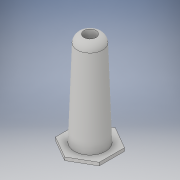
# Autodesk Inventor part: insert
Saved by Autodesk Inventor 2017 (Build 210142000, 142)
## iProperties
Created: 2017-08-01
Part Number: insert
Material: Generic
Document SubType Name: Modeling
Designer: Mitch
Density: 1 g/cm^3
Appearance: Default
Author: Mitch
Autodesk Inventor part; units mm, degrees
ref_plane "YZ Plane" through (0, 0, 0) normal (1, 0, 0) x (0, 1, 0)
ref_plane "XZ Plane" through (0, 0, 0) normal (0, 1, 0) x (-1, 0, 0)
sketch "Sketch1" plane through (0, 0, 0) normal (0, 1, 0) x (-1, 0, 0)
  line L0 (0, -10.2653) -> (-8.89, -5.1326)
  line L1 (-8.89, -5.1326) -> (-8.89, 5.1326)
  line L2 (-8.89, 5.1326) -> (0, 10.2653)
  line L3 (0, 10.2653) -> (8.89, 5.1326)
  line L4 (8.89, 5.1326) -> (8.89, -5.1326)
  line L5 (8.89, -5.1326) -> (0, -10.2653)
  point P0 (0, 0)
  point P1 (0, 0)
  dimension "d0" = 17.78
  constraints: 12 end point, 1 coincident, 13 other
  measures "d0" distance between parallel lines of L1 L4
extrude "Extrusion1" add sketch "Sketch1" along normal blind 1.27
sketch "Sketch2" plane through (0, 1.27, 0) normal (0, 1, 0) x (1, 0, 0)
  circle A0 centre (0, 0) radius 6.35
  dimension "d3" = 12.7
  constraints: 1 centre point, 1 coincident
  measures "d3" diameter of A0
ref_plane "Work Plane1" through (0, 39.37, 0) normal (0, 1, 0) x (1, 0, 0)
sketch "Sketch3" plane through (0, 39.37, 0) normal (0, 1, 0) x (1, 0, 0)
  circle A0 centre (0, 0) radius 5.08
  dimension "d5" = 10.16
  constraints: 1 centre point, 1 coincident
  measures "d5" diameter of A0
loft "Loft1" add profiles "Sketch2", "Sketch3"
fillet "Fillet1" radius 3.175 1 edges at (-5.08, 39.37, 0)
hole "Hole1" at (0, 39.37, 0) direction (0, -1, 0) diameter 4.953 depth 50.8 tip angle 118
body "Solid1"
